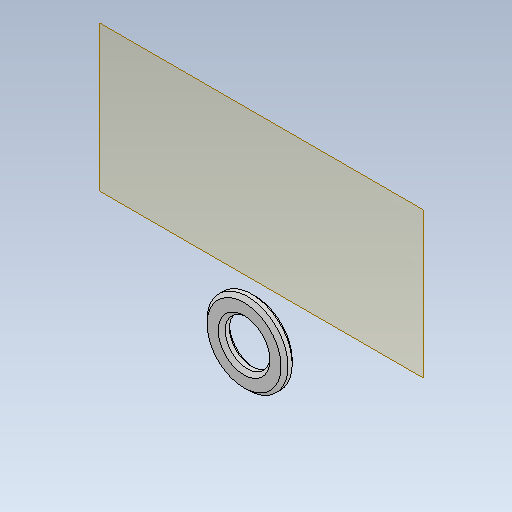
# Autodesk Inventor part: washers
Saved by Autodesk Inventor 2023 (Build 270158030, 158C)
## iProperties
Created: 2024-12-21
Part Number: washers
Material: Generic
Document SubType Name: Modeling
Designer: Imogen Heard
Density: 1 g/cm^3
Appearance: Default
Author: Imogen Heard
Autodesk Inventor part; units mm, degrees
ref_plane "YZ Plane" through (0, 0, 0) normal (1, 0, 0) x (0, 1, 0)
ref_plane "XZ Plane" through (0, 0, 0) normal (0, 1, 0) x (-1, 0, 0)
ref_plane "XY Plane" through (0, 0, 0) normal (0, 0, 1) x (1, 0, 0)
ref_plane "Work Plane1" through (0, 0, 0) normal (0, 0, 1) x (1, 0, 0)
sketch "Sketch1" plane through (0, 0, 0) normal (0, 0, 1) x (1, 0, 0)
  circle A0 centre (-0.9133, -5.3891) radius 4 projected
  circle A1 centre (-0.9133, -5.3891) radius 3.8536 projected
  circle A2 centre (-0.9133, -5.3891) radius 5.8
  circle A3 centre (-0.9133, -5.3891) radius 3.2
  point P0 (0, 0)
  dimension "d0" = 1.8
  dimension "d6" = 6.4
  constraints: 2 centre point
  measures "d0" radial gap between concentric circles of A2 A0
  measures "d6" diameter of A3
extrude "Extrusion1" add sketch "Sketch1" along normal blind 1.6 contours A0 | A1 | A2
chamfer "Chamfer1" distance 0.5 angle 45 2 edges at (-6.7133, -5.3891, 1.6) (-6.7133, -5.3891, 0)
chamfer "Chamfer2" distance 0.5 angle 45 2 edges at (-4.1133, -5.3891, 0) (-4.1133, -5.3891, 1.6)
